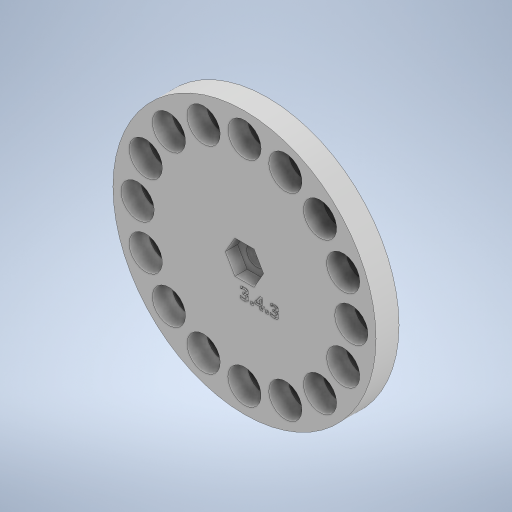
# Autodesk Inventor part: PancakeStator
Saved by Autodesk Inventor 2024.3 (Build 283343000, 343)
## iProperties
Created: 2024-11-27
Part Number: PancakeStator
Material: Generisch
Document SubType Name: Modeling
Designer: Maximilian Hock
Density: 1 g/cm^3
Appearance: Vorgabe
Author: Maximilian Hock
## iProperties of the stored document PancakeRotor_3D-Druck.ipt
Created: 2024-12-05
Part Number: PancakeRotor_3D-Druck
Material: Generisch
Document SubType Name: Modeling
Designer: Maximilian Hock
Density: 1 g/cm^3
Appearance: Vorgabe
Author: Maximilian Hock
Autodesk Inventor part; units mm, degrees
ref_plane "YZ Plane" through (0, 0, 0) normal (1, 0, 0) x (0, 1, 0)
ref_plane "XZ Plane" through (0, 0, 0) normal (0, 1, 0) x (-1, 0, 0)
ref_plane "XY Plane" through (0, 0, 0) normal (0, 0, 1) x (1, 0, 0)
sketch "Skizze1" plane through (0, 0, 0) normal (0, 1, 0) x (-1, 0, 0)
  circle A0 centre (0, 0) radius 40
  circle A1 centre (0, 0) radius 3.05
  dimension "d0" = 80
  dimension "d33" = 6.1
  constraints: 2 centre point, 2 coincident
  measures "d0" diameter of A0
  measures "d33" diameter of A1
extrude "Extrusion1" add sketch "Skizze1" against normal blind 7
sketch "Skizze3" plane through (0, -7, 0) normal (0, -1, 0) x (1, 0, 0)
  line L0 (-5.8235, 0) -> (-2.9118, 5.0433)
  line L1 (-2.9118, 5.0433) -> (2.9117, 5.0433)
  line L2 (2.9117, 5.0433) -> (5.8235, 0)
  line L3 (5.8235, 0) -> (2.9118, -5.0433)
  line L4 (2.9118, -5.0433) -> (-2.9117, -5.0433)
  line L5 (-2.9117, -5.0433) -> (-5.8235, 0)
  point P0 (0, 32.5)
  point P1 (0, 0)
  point P2 (0, 0)
  point P3 (0, 0)
  point P4 (0, 0)
  dimension "d24" = 32.5
  dimension "d38" = 11.647
  constraints: 12 end point, 3 coincident, 1 horizontal, 1 vertical alignment, 13 other
  measures "d24" distance of point (0, 0) point (0, 32.5)
  measures "d38" distance of L2.end L0.start
hole "Bohrung1" at (0, -7, 32.5) direction (0, 1, 0) diameter 7 end through all counterbore diameter 10.1 counterbore depth 6
pattern_circular "Runde Anordnung3" count 16 over 360 about axis through (0, -10, 0) along (0, 1, 0) of "Bohrung1"
extrude "Extrusion4" cut sketch "Skizze3" against normal blind 3.7
sketch "Skizze4" plane through (0, -7, 0) normal (0, -1, 0) x (1, 0, 0)
  line L0 (-2.9117, -5.0433) -> (12.2478, -5.0433) construction
  line L1 (12.2478, -5.0433) -> (12.2478, -11.5597) construction
  line L2 (12.2478, -11.5597) -> (-2.9117, -11.5597) construction
  line L3 (-2.9117, -11.5597) -> (-2.9117, -5.0433) construction
  spline S0 degree 2 poles (1.337, -8.9907) (1.337, -9.2488) (1.147, -9.6714) (0.9626, -9.8189) knots 0 0 0 1 2 2 2
  spline S1 degree 2 poles (0.9626, -9.8189) (0.7783, -9.9664) (0.2763, -10.1253) (-0.084, -10.1253) knots 0 0 0 1 2 2 2
  spline S2 degree 2 poles (-0.084, -10.1253) (-0.4924, -10.1253) (-1.0767, -9.9891) (-1.261, -9.904) knots 0 0 0 1 2 2 2
  line L4 (-1.261, -9.904) -> (-1.261, -9.1439)
  line L5 (-1.261, -9.1439) -> (-1.1759, -9.1439)
  spline S3 degree 2 poles (-1.1759, -9.1439) (-0.9831, -9.2659) (-0.464, -9.4474) (-0.2485, -9.4474) knots 0 0 0 1 2 2 2
  spline S4 degree 2 poles (-0.2485, -9.4474) (-0.1208, -9.4474) (0.177, -9.402) (0.2791, -9.3283) knots 0 0 0 1 2 2 2
  spline S5 degree 2 poles (0.2791, -9.3283) (0.3585, -9.2687) (0.4549, -9.0957) (0.4549, -8.9397) knots 0 0 0 1 2 2 2
  spline S6 degree 2 poles (0.4549, -8.9397) (0.4549, -8.7837) (0.3188, -8.6163) (0.2053, -8.5766) knots 0 0 0 1 2 2 2
  spline S7 degree 2 poles (0.2053, -8.5766) (0.0919, -8.5369) (-0.2229, -8.5284) (-0.3449, -8.5284) knots 0 0 0 1 2 2 2
  line L6 (-0.3449, -8.5284) -> (-0.4952, -8.5284)
  line L7 (-0.4952, -8.5284) -> (-0.4952, -7.9129)
  line L8 (-0.4952, -7.9129) -> (-0.3562, -7.9129)
  spline S8 degree 2 poles (-0.3562, -7.9129) (-0.1974, -7.9129) (0.072, -7.8846) (0.1656, -7.842) knots 0 0 0 1 2 2 2
  spline S9 degree 2 poles (0.1656, -7.842) (0.2592, -7.7966) (0.3642, -7.6378) (0.3642, -7.5017) knots 0 0 0 1 2 2 2
  spline S10 degree 2 poles (0.3642, -7.5017) (0.3642, -7.3939) (0.2649, -7.2606) (0.194, -7.2237) knots 0 0 0 1 2 2 2
  spline S11 degree 2 poles (0.194, -7.2237) (0.1089, -7.1812) (-0.118, -7.1528) (-0.1974, -7.1528) knots 0 0 0 1 2 2 2
  spline S12 degree 2 poles (-0.1974, -7.1528) (-0.325, -7.1528) (-0.5945, -7.2124) (-0.7193, -7.2606) knots 0 0 0 1 2 2 2
  spline S13 degree 2 poles (-0.7193, -7.2606) (-0.8186, -7.2975) (-1.0341, -7.4166) (-1.0852, -7.4478) knots 0 0 0 1 2 2 2
  line L9 (-1.0852, -7.4478) -> (-1.1589, -7.4478)
  line L10 (-1.1589, -7.4478) -> (-1.1589, -6.699)
  spline S14 degree 2 poles (-1.1589, -6.699) (-0.9774, -6.6224) (-0.3647, -6.4778) (-0.0442, -6.4778) knots 0 0 0 1 2 2 2
  spline S15 degree 2 poles (-0.0442, -6.4778) (0.2677, -6.4778) (0.7272, -6.5855) (0.8889, -6.6905) knots 0 0 0 1 2 2 2
  spline S16 degree 2 poles (0.8889, -6.6905) (1.0676, -6.8011) (1.2463, -7.1415) (1.2463, -7.3542) knots 0 0 0 1 2 2 2
  spline S17 degree 2 poles (1.2463, -7.3542) (1.2463, -7.6548) (0.9002, -8.103) (0.6166, -8.1682) knots 0 0 0 1 2 2 2
  line L11 (0.6166, -8.1682) -> (0.6166, -8.2022)
  spline S18 degree 2 poles (0.6166, -8.2022) (0.7414, -8.2193) (0.9797, -8.31) (1.0931, -8.4121) knots 0 0 0 1 2 2 2
  spline S19 degree 2 poles (1.0931, -8.4121) (1.1981, -8.5029) (1.337, -8.7922) (1.337, -8.9907) knots 0 0 0 1 2 2 2
  line L12 (2.7297, -10.0515) -> (1.8986, -10.0515)
  line L13 (1.8986, -10.0515) -> (1.8986, -9.1269)
  line L14 (1.8986, -9.1269) -> (2.7297, -9.1269)
  line L15 (2.7297, -9.1269) -> (2.7297, -10.0515)
  line L16 (6.0368, -9.2347) -> (5.5631, -9.2347)
  line L17 (5.5631, -9.2347) -> (5.5631, -10.06)
  line L18 (5.5631, -10.06) -> (4.7151, -10.06)
  line L19 (4.7151, -10.06) -> (4.7151, -9.2347)
  line L20 (4.7151, -9.2347) -> (3.1721, -9.2347)
  line L21 (3.1721, -9.2347) -> (3.1721, -8.5823)
  line L22 (3.1721, -8.5823) -> (4.6867, -6.5515)
  line L23 (4.6867, -6.5515) -> (5.5631, -6.5515)
  line L24 (5.5631, -6.5515) -> (5.5631, -8.605)
  line L25 (5.5631, -8.605) -> (6.0368, -8.605)
  line L26 (6.0368, -8.605) -> (6.0368, -9.2347)
  line L27 (4.7151, -8.605) -> (4.7151, -7.4137)
  line L28 (4.7151, -7.4137) -> (3.8273, -8.605)
  line L29 (3.8273, -8.605) -> (4.7151, -8.605)
  line L30 (7.2989, -10.0515) -> (6.4679, -10.0515)
  line L31 (6.4679, -10.0515) -> (6.4679, -9.1269)
  line L32 (6.4679, -9.1269) -> (7.2989, -9.1269)
  line L33 (7.2989, -9.1269) -> (7.2989, -10.0515)
  spline S20 degree 2 poles (10.4756, -8.9907) (10.4756, -9.2488) (10.2856, -9.6714) (10.1012, -9.8189) knots 0 0 0 1 2 2 2
  spline S21 degree 2 poles (10.1012, -9.8189) (9.9169, -9.9664) (9.4148, -10.1253) (9.0546, -10.1253) knots 0 0 0 1 2 2 2
  spline S22 degree 2 poles (9.0546, -10.1253) (8.6462, -10.1253) (8.0619, -9.9891) (7.8776, -9.904) knots 0 0 0 1 2 2 2
  line L34 (7.8776, -9.904) -> (7.8776, -9.1439)
  line L35 (7.8776, -9.1439) -> (7.9626, -9.1439)
  spline S23 degree 2 poles (7.9626, -9.1439) (8.1555, -9.2659) (8.6746, -9.4474) (8.8901, -9.4474) knots 0 0 0 1 2 2 2
  spline S24 degree 2 poles (8.8901, -9.4474) (9.0177, -9.4474) (9.3156, -9.402) (9.4177, -9.3283) knots 0 0 0 1 2 2 2
  spline S25 degree 2 poles (9.4177, -9.3283) (9.4971, -9.2687) (9.5935, -9.0957) (9.5935, -8.9397) knots 0 0 0 1 2 2 2
  spline S26 degree 2 poles (9.5935, -8.9397) (9.5935, -8.7837) (9.4574, -8.6163) (9.3439, -8.5766) knots 0 0 0 1 2 2 2
  spline S27 degree 2 poles (9.3439, -8.5766) (9.2305, -8.5369) (8.9156, -8.5284) (8.7937, -8.5284) knots 0 0 0 1 2 2 2
  line L36 (8.7937, -8.5284) -> (8.6434, -8.5284)
  line L37 (8.6434, -8.5284) -> (8.6434, -7.9129)
  line L38 (8.6434, -7.9129) -> (8.7823, -7.9129)
  spline S28 degree 2 poles (8.7823, -7.9129) (8.9412, -7.9129) (9.2106, -7.8846) (9.3042, -7.842) knots 0 0 0 1 2 2 2
  spline S29 degree 2 poles (9.3042, -7.842) (9.3978, -7.7966) (9.5028, -7.6378) (9.5028, -7.5017) knots 0 0 0 1 2 2 2
  spline S30 degree 2 poles (9.5028, -7.5017) (9.5028, -7.3939) (9.4035, -7.2606) (9.3326, -7.2237) knots 0 0 0 1 2 2 2
  spline S31 degree 2 poles (9.3326, -7.2237) (9.2475, -7.1812) (9.0206, -7.1528) (8.9412, -7.1528) knots 0 0 0 1 2 2 2
  spline S32 degree 2 poles (8.9412, -7.1528) (8.8135, -7.1528) (8.5441, -7.2124) (8.4193, -7.2606) knots 0 0 0 1 2 2 2
  spline S33 degree 2 poles (8.4193, -7.2606) (8.32, -7.2975) (8.1045, -7.4166) (8.0534, -7.4478) knots 0 0 0 1 2 2 2
  line L39 (8.0534, -7.4478) -> (7.9797, -7.4478)
  line L40 (7.9797, -7.4478) -> (7.9797, -6.699)
  spline S34 degree 2 poles (7.9797, -6.699) (8.1612, -6.6224) (8.7738, -6.4778) (9.0943, -6.4778) knots 0 0 0 1 2 2 2
  spline S35 degree 2 poles (9.0943, -6.4778) (9.4063, -6.4778) (9.8658, -6.5855) (10.0275, -6.6905) knots 0 0 0 1 2 2 2
  spline S36 degree 2 poles (10.0275, -6.6905) (10.2062, -6.8011) (10.3848, -7.1415) (10.3848, -7.3542) knots 0 0 0 1 2 2 2
  spline S37 degree 2 poles (10.3848, -7.3542) (10.3848, -7.6548) (10.0388, -8.103) (9.7552, -8.1682) knots 0 0 0 1 2 2 2
  line L41 (9.7552, -8.1682) -> (9.7552, -8.2022)
  spline S38 degree 2 poles (9.7552, -8.2022) (9.88, -8.2193) (10.1182, -8.31) (10.2317, -8.4121) knots 0 0 0 1 2 2 2
  spline S39 degree 2 poles (10.2317, -8.4121) (10.3366, -8.5029) (10.4756, -8.7922) (10.4756, -8.9907) knots 0 0 0 1 2 2 2
  point P0 (0, 0)
  point P1 (-2.9117, -5.0433)
  constraints: 1 coincident, 2 other
emboss "Prägen1" sketch "Skizze4" operation cut depth 0.5 direction (0, 1, 0)
equation "\"d0\" = RotorDiameter"
equation "\"d33\" = AxleDiameter + Clearance"
equation "\"d1\" = RotorThickness"
equation "\"d24\" = MagnetDistance"
equation "\"d38\" = HexnutOuterSize + Clearance"
equation "\"d11\" = MagnetDiameter + Clearance"
equation "\"d12\" = 2 * MagnetHeight"
equation "\"d14\" = MagnetHeight"
equation "\"d35\" = HexnutHeight - Airgap"
equation "\"StatorThickness\" = 3"
equation "\"RotorDiameter\" = 80"
equation "\"AxleDiameter\" = 6"
equation "\"Clearance\" = 0.1"
equation "\"RotorThickness\" = 7"
equation "\"HexnutOuterSize\" = 11.547"
equation "\"MagnetDiameter\" = 10"
equation "\"MagnetHeight\" = 3"
equation "\"HexnutHeight\" = 4.7"
equation "\"Airgap\" = 1"
equation "\"MagnetDistance\" = 32.5"
